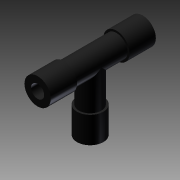
# Autodesk Inventor part: Joiner Base 1764
Saved by Autodesk Inventor 2011 (Build 150239000, 239)
## iProperties
Created: 2010-02-21
Part Number: Joiner Base 1764
Document SubType Name: Modeling
Designer: jgehrig
Density: 1 g/cm^3
Author: jgehrig
Autodesk Inventor part; units mm, degrees
ref_plane "YZ Plane" through (0, 0, 0) normal (1, 0, 0) x (0, 1, 0)
sketch "Sketch1" plane through (0, 0, 0) normal (0, 0, 1) x (1, 0, 0)
  circle A0 centre (-21.4074, 14.2963) radius 6.35
  circle A1 centre (-21.4074, 14.2963) radius 3.175
  point P0 (0, 0)
  dimension "d0" = 12.7
  dimension "d1" = 6.35
  constraints: 2 centre point, 1 coincident
  measures "d0" diameter of A0
  measures "d1" diameter of A1
extrude "Extrusion1" add sketch "Sketch1" along normal blind 12.7
sketch "Sketch2" plane through (-21.4074, 14.2963, 0) normal (0, 0, -1) x (-1, 0, 0)
  circle A0 centre (0, 0) radius 3.175 projected
  circle A1 centre (0, 0) radius 6.35 projected
  circle A2 centre (0, 0) radius 5.3975
  point P0 (-21.4074, -14.2963)
  dimension "d4" = 10.795
  constraints: 1 centre point, 1 coincident
  measures "d4" diameter of A2
extrude "Extrusion2" add sketch "Sketch2" along normal blind 25.4 contours A2
sketch "Sketch3" plane through (-21.4074, 14.2963, -25.4) normal (0, 0, -1) x (-1, 0, 0)
  circle A0 centre (0, 0) radius 3.175 projected
  circle A1 centre (0, 0) radius 5.3975 projected
  circle A2 centre (0, 0) radius 6.35
  point P0 (-21.4074, -14.2963)
  dimension "d7" = 12.7
  constraints: 1 centre point, 1 coincident
  measures "d7" diameter of A2
extrude "Extrusion3" add sketch "Sketch3" along normal blind 12.7 contours A1 | A2
ref_plane "Work Plane3" through (0, 19.685, 0) normal (0, 1, 0) x (-1, 0, 0)
sketch "Sketch4" plane through (0, 19.685, 0) normal (0, 1, 0) x (-1, 0, 0)
  line L0 (26.8049, -25.4) -> (16.0099, -25.4) projected
  line L1 (26.8049, 0) -> (16.0099, 0) projected
  line L2 (26.8049, 0) -> (26.8049, -25.4) projected
  line L3 (16.0099, 0) -> (16.0099, -25.4) projected
  circle A0 centre (21.4074, -12.7) radius 5.3975
  circle A1 centre (21.4074, -12.7) radius 3.175
  point P0 (0, 0)
  dimension "d13" = 6.35
  constraints: 2 centre point, 1 coincident, 1 tangent
  measures "d13" diameter of A1
extrude "Extrusion4" add sketch "Sketch4" against normal blind 23.495 contours A0
sketch "Sketch5" plane through (-21.4074, -3.81, -12.7) normal (0, -1, 0) x (1, 0, 0)
  circle A0 centre (0, 0) radius 3.175 projected
  circle A1 centre (0, 0) radius 5.3975 projected
  circle A2 centre (0, 0) radius 6.35
  point P0 (21.4074, 12.7)
  dimension "d16" = 12.7
  constraints: 1 centre point, 1 coincident
  measures "d16" diameter of A2
extrude "Extrusion5" add sketch "Sketch5" along normal blind 12.7 contours A1 | A2
ref_plane "Work Plane5" through (0, 0, 0) normal (0, 0, 1) x (1, 0, 0)
sketch "Sketch7" plane through (0, 0, 0) normal (0, 0, 1) x (1, 0, 0)
  circle A0 centre (-21.4074, 14.2963) radius 5.3975 projected
  circle A1 centre (-21.4074, 14.2963) radius 5.3975
  line L0 (-16.0099, 19.6938) -> (-26.8049, 19.6938)
  line L1 (-26.8049, 19.6938) -> (-26.8049, 8.8988)
  line L2 (-26.8049, 8.8988) -> (-16.0099, 8.8988)
  line L3 (-16.0099, 8.8988) -> (-16.0099, 19.6938)
  line L4 (-16.0099, 14.2963) -> (-26.8049, 14.2963)
  line L5 (-16.0099, 14.2963) -> (-26.8049, 14.2963)
  line L6 (-26.8049, 14.2963) -> (-26.8049, 8.8988)
  line L7 (-26.8049, 8.8988) -> (-16.0099, 8.8988)
  line L8 (-16.0099, 8.8988) -> (-16.0099, 14.2963)
  arc A2 (-26.8049, 14.2963) -> (-16.0099, 14.2963) centre (-21.4074, 14.2963) ccw
  line L9 (-16.0099, 19.6938) -> (-26.8049, 19.6938)
  line L10 (-26.8049, 19.6938) -> (-26.8049, 14.2963)
  line L11 (-26.8049, 14.2963) -> (-16.0099, 14.2963)
  line L12 (-16.0099, 14.2963) -> (-16.0099, 19.6938)
  arc A3 (-16.0099, 14.2963) -> (-26.8049, 14.2963) centre (-21.4074, 14.2963) ccw
  point P0 (0, 0)
  constraints: 26 end point, 6 parallel, 4 point on circle, 4 tangent, 3 centre point, 3 horizontal, 3 perpendicular, 2 midpoint, 1 coincident, 1 concentric
extrude "Extrusion7" cut sketch "Sketch7" against normal blind 25.4 contours A0 L0 L3 | A0 L1 L0
body "Solid1"
